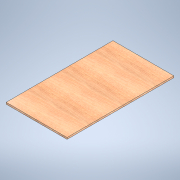
# Autodesk Inventor part: baseForLongRobot
Saved by Autodesk Inventor 2020.2 (Build 242310000, 310)
## iProperties
Created: 2020-01-09
Part Number: baseForLongRobot
Material: Wood (Birch)
Document SubType Name: Modeling
Designer: steele
Density: 0.55 g/cm^3
Appearance: Birch - Natural Polished
Author: steele
Autodesk Inventor part; units mm, degrees
ref_plane "YZ Plane" through (0, 0, 0) normal (1, 0, 0) x (0, 1, 0)
ref_plane "XZ Plane" through (0, 0, 0) normal (0, 1, 0) x (-1, 0, 0)
ref_plane "XY Plane" through (0, 0, 0) normal (0, 0, 1) x (1, 0, 0)
sketch "Sketch1" plane through (0, 0, 0) normal (0, 1, 0) x (-1, 0, 0)
  line L0 (231.775, 406.4) -> (-231.775, 406.4)
  line L1 (-231.775, 406.4) -> (-231.775, -406.4)
  line L2 (-231.775, -406.4) -> (231.775, -406.4)
  line L3 (231.775, -406.4) -> (231.775, 406.4)
  line L4 (231.775, 406.4) -> (-231.775, -406.4) construction
  line L5 (-231.775, 406.4) -> (231.775, -406.4) construction
  point P0 (0, 0)
  dimension "d0" = 463.55
  dimension "d1" = 812.8
  constraints: 12 end point, 2 midpoint, 2 parallel, 1 horizontal, 1 perpendicular
  measures "d0" distance of L0.start L0.end
  measures "d1" distance of L1.end L0.end
extrude "Extrusion1" add sketch "Sketch1" along normal blind 12.7
body "Solid1"
